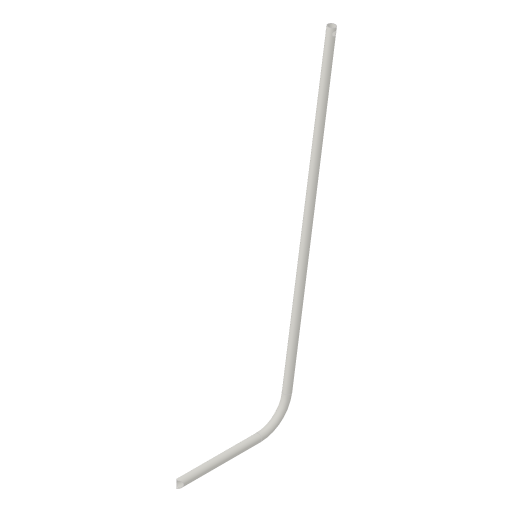
# Autodesk Inventor part: Hebel
Saved by Autodesk Inventor 2023.2 (Build 272271000, 271)
## iProperties
Created: 2023-02-02
Part Number: Hebel
Material: Stahl ASTM A36
Document SubType Name: Modeling
Designer: Raoul Messerli
Density: 7.85 g/cm^3
Appearance: Schweißnaht - Stahl - weich
Mass: 33018.3 g
Surface Area: 22315.8 cm^2
Volume: 4206.15 cm^3
Author: Raoul Messerli
Autodesk Inventor part; units mm, degrees
ref_plane "YZ Plane" through (0, 0, 0) normal (1, 0, 0) x (0, 1, 0)
ref_plane "XY Plane" through (0, 0, 0) normal (0, 0, 1) x (1, 0, 0)
sketch "Skizze2" plane through (0, 0, 0) normal (1, 0, 0) x (0, 1, 0)
  line L0 (0, 0) -> (842.0372, 0)
  arc A0 (842.0372, 0) -> (1138.6507, 255.0509) centre (842.0372, 300) ccw
  line L1 (1138.6507, 255.0509) -> (1600, 3299.4356)
  line L2 (1138.6507, 255.0509) -> (1100, 0)
  line L3 (842.0372, 0) -> (1100, 0)
  point P0 (1592.5085, 3250)
  dimension "d6" = 300
  dimension "d7" = 1600
  dimension "d18" = 1100
  dimension "d37" = 98.617
  dimension "d38" = 50
  dimension "d41" = 3337.1058
  dimension "d42" = 3250
  constraints: 8 end point, 3 tangent, 2 horizontal, 2 point on circle, 1 centre point, 1 coincident, 1 point on line
  measures "d6" radius of A0
  measures "d7" horizontal distance of L0.start L1.end
  measures "d18" distance of L0.start L2.end
  measures "d37" angle of L0 L1
  measures "d38" distance of L1.end point (1592.508, 3250)
  measures "d41" distance of L2.end L1.end
  measures "d42" distance from line of L0 point (1592.508, 3250)
sketch "Skizze3" plane through (0, 0, 0) normal (0, 1, 0) x (-1, 0, 0)
  circle A0 centre (0, 0) radius 38.05
  circle A1 centre (0, 0) radius 34.45
  dimension "d12" = 76.1
  dimension "d13" = 3.6
  constraints: 2 centre point, 2 coincident
  measures "d12" diameter of A0
  measures "d13" radial gap between concentric circles of A1 A0
sweep "Sweeping1" add profiles "Skizze3" path "Skizze2" path curves L0 A0 L1
sketch "Skizze5" plane through (0, 0, 0) normal (1, 0, 0) x (0, 1, 0)
  line L0 (0, -38.05) -> (0, 38.05) projected
  circle A0 centre (0, 0) radius 38.05
  constraints: 1 coincident, 1 vertical alignment, 2 other
extrude "Extrusion3" cut sketch "Skizze5" along normal mid plane 76.1
sketch "Skizze6" plane through (0, 0, 0) normal (1, 0, 0) x (0, 1, 0)
  line L0 (1637.6205, 3293.7345) -> (1562.3795, 3305.1366) projected
  line L1 (1600, 3299.4356) -> (1592.5085, 3250)
  circle A0 centre (1592.5085, 3250) radius 21.5
  point P0 (0, 0)
  dimension "d19" = 43
  dimension "d21" = 50
  constraints: 2 end point, 1 centre point, 1 coincident, 1 midpoint, 1 perpendicular
  measures "d19" diameter of A0
  measures "d21" distance of L1.start L1.end
extrude "Extrusion4" cut sketch "Skizze6" along normal through all both and the other way through all
ref_plane "Arbeitsebene1" through (0, 1715, 0) normal (0, 1, 0) x (-1, 0, 0)
